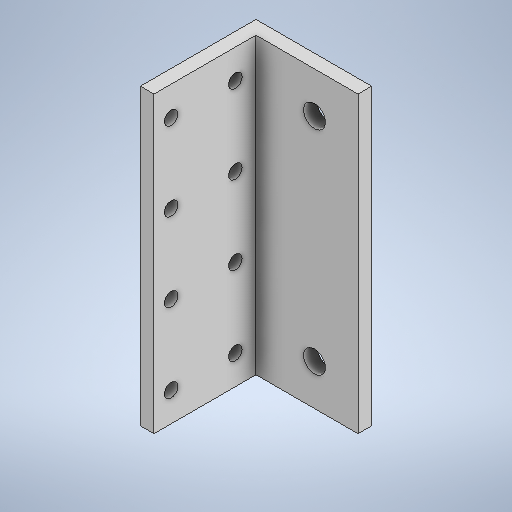
# Autodesk Inventor part: MuteMount
Saved by Autodesk Inventor 2025.1 (Build 291241000, 241)
## iProperties
Created: 2025-12-01
Part Number: MuteMount
Material: Generic
Document SubType Name: Modeling
Designer: Juxin
Density: 1 g/cm^3
Appearance: Default
Author: Juxin
Autodesk Inventor part; units mm, degrees
ref_plane "YZ Plane" through (0, 0, 0) normal (1, 0, 0) x (0, 1, 0)
ref_plane "XZ Plane" through (0, 0, 0) normal (0, 1, 0) x (-1, 0, 0)
ref_plane "XY Plane" through (0, 0, 0) normal (0, 0, 1) x (1, 0, 0)
sketch "Sketch1" plane through (0, 0, 0) normal (0, 1, 0) x (-1, 0, 0)
  line L0 (0, 0) -> (26.9875, 0)
  line L1 (26.9875, 0) -> (26.9875, -26.9875)
  line L2 (26.9875, -26.9875) -> (0, -26.9875)
  line L3 (0, -26.9875) -> (0, 0)
  line L4 (26.9875, -23.3392) -> (23.8125, -23.3392)
  line L5 (0, -23.8125) -> (0, 0)
  line L6 (0, 0) -> (51.181, 0)
  line L7 (23.8125, -26.9875) -> (23.8125, -23.8125)
  line L8 (23.8125, -23.8125) -> (0, -23.8125)
  line L9 (0, -23.8125) -> (0, 0)
  line L10 (0, 0) -> (23.8125, 0)
  line L11 (23.8125, 0) -> (23.8125, -23.8125)
  dimension "d0" = 26.9875
  dimension "d1" = 26.9875
  dimension "d2" = 3.175
  dimension "d4" = 3.175
  constraints: 24 end point, 4 parallel, 3 horizontal, 2 perpendicular, 2 point on line, 1 vertical
  measures "d0" distance of L1.end L2.end
  measures "d1" distance of L0.end L1.end
  measures "d2" distance of L4.start L4.end
  measures "d4" distance of L7.start L7.end
extrude "Extrusion1" add sketch "Sketch1" along normal blind 18.3642 contours L0 L1 L4 L11 | L8 L7 L2 L3 | L4 L1 L2 L7 L11
sketch "Sketch4" plane through (-26.9875, 0, -26.9875) normal (-1, 0, 0) x (0, 0, 1)
  line L0 (26.9875, 0) -> (26.9875, 18.3642) projected
  line L1 (0, 0) -> (26.9875, 0)
  line L2 (26.9875, 0) -> (26.9875, 13.589)
  line L3 (26.9875, 13.589) -> (0, 13.589)
  line L4 (0, 13.589) -> (0, 0)
  line L5 (0, 0) -> (0, 18.3642) projected
  line L6 (0, 6.7945) -> (8.001, 6.7945)
  circle A0 centre (8.001, 6.7945) radius 1.5875
  line L7 (8.001, 6.7945) -> (22.987, 6.7945)
  circle A1 centre (22.987, 6.7945) radius 1.5875
  dimension "d23" = 13.589
  dimension "d24" = 8.001
  dimension "d25" = 3.175
  dimension "d26" = 14.986
  dimension "d27" = 3.175
  constraints: 12 end point, 2 centre point, 2 coincident, 2 horizontal, 2 parallel, 2 perpendicular, 2 point on line
  measures "d23" distance of L2.end L1.end
  measures "d24" distance of L6.start L6.end
  measures "d25" diameter of A0
  measures "d26" distance of L7.start L7.end
  measures "d27" diameter of A1
extrude "Extrusion4" cut sketch "Sketch4" against normal blind 18.3642 contours A0 L7 L6 | L6 L7 A0 | A1
move faces "Move1" translate (0, 13.589, 0) faces at (-16.9333, 18.3642, -25.9292)
sketch "Sketch5" plane through (-26.9875, 0, -26.9875) normal (-1, 0, 0) x (0, 0, 1)
  line L0 (26.9875, 0) -> (26.9875, 31.9532) projected
  line L1 (0, 0) -> (0, 31.9532) projected
  line L2 (26.9875, 31.9532) -> (0, 31.9532)
  line L3 (0, 31.9532) -> (0, 18.3642)
  line L4 (0, 18.3642) -> (26.9875, 18.3642)
  line L5 (26.9875, 18.3642) -> (26.9875, 31.9532)
  line L6 (0, 25.1587) -> (8.001, 25.1587)
  circle A0 centre (8.001, 25.1587) radius 1.5875
  line L7 (8.001, 25.1587) -> (22.987, 25.1587)
  circle A1 centre (22.987, 25.1587) radius 1.5875
  dimension "d33" = 13.589
  dimension "d34" = 8.001
  dimension "d35" = 3.175
  dimension "d36" = 14.986
  dimension "d37" = 3.175
  constraints: 12 end point, 3 horizontal, 2 centre point, 2 coincident, 2 parallel, 1 midpoint, 1 perpendicular, 1 point on line
  measures "d33" distance of L3.end L2.end
  measures "d34" distance of L6.start L6.end
  measures "d35" diameter of A0
  measures "d36" distance of L7.start L7.end
  measures "d37" diameter of A1
extrude "Extrusion5" cut sketch "Sketch5" against normal blind 18.3642 contours A0 L7 L6 | L6 L7 A0 | A1
move faces "Move2" translate (0, 18.3515, 0) faces at (-16.9333, 31.9532, -25.9292)
sketch "Sketch6" plane through (-26.9875, 0, -26.9875) normal (-1, 0, 0) x (0, 0, 1)
  line L0 (26.9875, 0) -> (26.9875, 50.3047) projected
  line L1 (0, 0) -> (0, 50.3047) projected
  line L2 (26.9875, 50.3047) -> (0, 50.3047)
  line L3 (0, 50.3047) -> (0, 36.7157)
  line L4 (0, 36.7157) -> (26.9875, 36.7157)
  line L5 (26.9875, 36.7157) -> (26.9875, 50.3047)
  line L6 (0, 43.5102) -> (8.001, 43.5102)
  circle A0 centre (8.001, 43.5102) radius 1.5875
  line L7 (8.001, 43.5102) -> (22.987, 43.5102)
  circle A1 centre (22.987, 43.5102) radius 1.5875
  dimension "d43" = 13.589
  dimension "d44" = 8.001
  dimension "d45" = 3.175
  dimension "d46" = 14.986
  dimension "d47" = 3.175
  constraints: 12 end point, 3 parallel, 2 centre point, 2 coincident, 2 horizontal, 1 midpoint, 1 perpendicular, 1 point on line
  measures "d43" distance of L3.end L2.end
  measures "d44" distance of L6.start L6.end
  measures "d45" diameter of A0
  measures "d46" distance of L7.start L7.end
  measures "d47" diameter of A1
extrude "Extrusion6" cut sketch "Sketch6" against normal blind 18.3642 contours A0 L7 L6 | L6 L7 A0 | A1
move faces "Move3" translate (0, 18.3515, 0) faces at (-16.9333, 50.3047, -25.9292)
sketch "Sketch7" plane through (-26.9875, 0, -26.9875) normal (-1, 0, 0) x (0, 0, 1)
  line L0 (26.9875, 0) -> (26.9875, 68.6562) projected
  line L1 (0, 0) -> (0, 68.6562) projected
  line L2 (26.9875, 68.6562) -> (0, 68.6562)
  line L3 (0, 68.6562) -> (0, 55.0672)
  line L4 (0, 55.0672) -> (26.9875, 55.0672)
  line L5 (26.9875, 55.0672) -> (26.9875, 68.6562)
  line L6 (0, 61.8617) -> (8.001, 61.8617)
  circle A0 centre (8.001, 61.8617) radius 1.5875
  line L7 (8.001, 61.8617) -> (22.987, 61.8617)
  circle A1 centre (22.987, 61.8617) radius 1.5875
  dimension "d53" = 13.589
  dimension "d54" = 8.001
  dimension "d55" = 3.175
  dimension "d56" = 14.986
  dimension "d57" = 3.175
  constraints: 12 end point, 3 horizontal, 2 centre point, 2 coincident, 2 parallel, 1 midpoint, 1 perpendicular, 1 point on line
  measures "d53" distance of L3.end L2.end
  measures "d54" distance of L6.start L6.end
  measures "d55" diameter of A0
  measures "d56" distance of L7.start L7.end
  measures "d57" diameter of A1
extrude "Extrusion7" cut sketch "Sketch7" against normal blind 18.3642 contours A0 L7 L6 | L6 L7 A0 | A1
sketch "Sketch8" plane through (0, 0, -26.9875) normal (0, 0, -1) x (-1, 0, 0)
  line L0 (0, 0) -> (0, 68.6562) projected
  line L1 (23.8125, 0) -> (0, 0) projected
  line L2 (0, 68.6562) -> (20.32, 68.6562)
  line L3 (20.32, 68.6562) -> (20.32, 0)
  line L4 (20.32, 0) -> (0, 0)
  line L5 (0, 0) -> (0, 68.6562)
  line L6 (10.16, 0) -> (10.16, 9.525)
  line L7 (10.16, 68.6562) -> (10.16, 59.1312)
  circle A0 centre (10.16, 59.1312) radius 2.54
  circle A1 centre (10.16, 9.525) radius 2.54
  dimension "d60" = 20.32
  dimension "d61" = 9.525
  dimension "d62" = 9.525
  dimension "d63" = 5.08
  dimension "d64" = 5.08
  constraints: 12 end point, 2 centre point, 2 coincident, 2 midpoint, 2 parallel, 2 vertical, 1 horizontal, 1 perpendicular, 1 point on line
  measures "d60" distance of L3.end L4.end
  measures "d61" distance of L6.start L6.end
  measures "d62" distance of L7.start L7.end
  measures "d63" diameter of A0
  measures "d64" diameter of A1
extrude "Extrusion8" cut sketch "Sketch8" against normal blind 18.3642 contours A0 | A1
body "Solid1"
